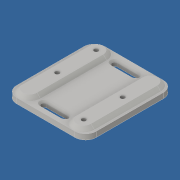
# Autodesk Inventor part: wandler
Saved by Autodesk Inventor 2016 (Build 200138000, 138)
## iProperties
Created: 2015-10-23
Part Number: wandler
Material: Generisch
Document SubType Name: Modeling
Designer: 4ndreas
Density: 1 g/cm^3
Appearance: Vorgabe
Author: 4ndreas
Autodesk Inventor part; units mm, degrees
ref_plane "YZ Plane" through (0, 0, 0) normal (1, 0, 0) x (0, 1, 0)
ref_plane "XZ Plane" through (0, 0, 0) normal (0, 1, 0) x (-1, 0, 0)
ref_plane "XY Plane" through (0, 0, 0) normal (0, 0, 1) x (1, 0, 0)
sketch "Skizze1" plane through (0, 0, 0) normal (0, 0, 1) x (1, 0, 0)
  line L0 (-22.5, -25) -> (22.5, -25)
  line L1 (22.5, -25) -> (22.5, 25)
  line L2 (22.5, 25) -> (-22.5, 25)
  line L3 (-22.5, 25) -> (-22.5, -25)
  line L4 (-22.5, -25) -> (22.5, 25) construction
  line L5 (22.5, -25) -> (-22.5, 25) construction
  line L6 (0, 11) -> (0, -11) construction
  line L7 (-15.25, 18.75) -> (15.25, 18.75) construction
  line L8 (15.25, 18.75) -> (15.25, 3.25) construction
  line L9 (15.25, 3.25) -> (-15.25, 3.25) construction
  line L10 (-15.25, 3.25) -> (-15.25, 18.75) construction
  line L11 (-15.25, 18.75) -> (15.25, 3.25) construction
  line L12 (15.25, 18.75) -> (-15.25, 3.25) construction
  line L13 (-17.7097, 20) -> (17.7097, 20) construction
  line L14 (17.7097, 20) -> (17.7097, 2) construction
  line L15 (17.7097, 2) -> (-17.7097, 2) construction
  line L16 (-17.7097, 2) -> (-17.7097, 20) construction
  line L17 (-17.7097, 20) -> (17.7097, 2) construction
  line L18 (17.7097, 20) -> (-17.7097, 2) construction
  line L19 (-15.25, -18.75) -> (15.25, -18.75) construction
  line L20 (15.25, -18.75) -> (15.25, -3.25) construction
  line L21 (15.25, -3.25) -> (-15.25, -3.25) construction
  line L22 (-15.25, -3.25) -> (-15.25, -18.75) construction
  line L23 (-15.25, -18.75) -> (15.25, -3.25) construction
  line L24 (15.25, -18.75) -> (-15.25, -3.25) construction
  circle A0 centre (-15.25, 18.75) radius 1.25
  circle A1 centre (15.25, 3.25) radius 1.25
  circle A2 centre (15.25, -18.75) radius 1.25
  circle A3 centre (-15.25, -3.25) radius 1.25
  point P0 (0, 0)
  point P1 (0, 0)
  dimension "d0" = 45
  dimension "d1" = 15.5
  dimension "d2" = 30.5
  dimension "d3" = 2
  dimension "d4" = 18
  dimension "d5" = 25
  dimension "d6" = 2.5
  constraints: 50 end point, 10 midpoint, 9 parallel, 7 coincident, 4 centre point, 4 horizontal, 4 perpendicular, 3 equal radius, 3 point on line, 2 equal length
  measures "d0" distance between parallel lines of L3 L1
  measures "d1" distance between parallel lines of L9 L7
  measures "d2" distance between parallel lines of L8 L10
  measures "d3" distance from line of point (0, 0) L15
  measures "d4" distance between parallel lines of L15 L13
  measures "d5" distance from line of point (0, 0) L2
  measures "d6" diameter of A0
extrude "Extrusion1" add sketch "Skizze1" along normal blind 3
fillet "Rundung1" radius 6 4 edges at (-22.5, 25, 1.5) (-22.5, -25, 1.5) (22.5, -25, 1.5) (22.5, 25, 1.5)
chamfer "Fase1" distance 2 angle 45 4 edges at (-16.5, -3.25, 0) (14, -18.75, 0) (14, 3.25, 0) (-16.5, 18.75, 0)
sketch "Skizze2" plane through (0, 0, 3) normal (0, 0, 1) x (1, 0, 0)
  arc A0 (22.5, 19) -> (16.5, 25) centre (16.5, 19) ccw projected
  line L0 (16.5, 25) -> (-16.5, 25) projected
  arc A1 (-16.5, 25) -> (-22.5, 19) centre (-16.5, 19) ccw projected
  line L1 (-22.5, 19) -> (-22.5, -19) projected
  arc A2 (-22.5, -19) -> (-16.5, -25) centre (-16.5, -19) ccw projected
  line L2 (-16.5, -25) -> (16.5, -25) projected
  arc A3 (16.5, -25) -> (22.5, -19) centre (16.5, -19) ccw projected
  line L3 (22.5, -19) -> (22.5, 19) projected
  circle A4 centre (-15.25, -3.25) radius 1.25 projected
  circle A5 centre (15.25, -18.75) radius 1.25 projected
  circle A6 centre (15.25, 3.25) radius 1.25 projected
  circle A7 centre (-15.25, 18.75) radius 1.25 projected
  circle A8 centre (15.25, 3.25) radius 4
  circle A9 centre (15.25, -18.75) radius 4
  circle A10 centre (-15.25, -3.25) radius 4
  circle A11 centre (-15.25, 18.75) radius 4
  line L4 (15.25, -18.75) -> (15.25, 18.75) construction
  line L5 (19.25, -18.75) -> (19.25, 18.75)
  line L6 (11.25, 18.75) -> (11.25, -18.75)
  arc A12 (11.25, -18.75) -> (19.25, -18.75) centre (15.25, -18.75) ccw
  arc A13 (19.25, 18.75) -> (11.25, 18.75) centre (15.25, 18.75) ccw
  line L7 (-15.25, 18.75) -> (-15.25, -18.75) construction
  line L8 (-19.25, 18.75) -> (-19.25, -18.75)
  line L9 (-11.25, -18.75) -> (-11.25, 18.75)
  arc A14 (-11.25, 18.75) -> (-19.25, 18.75) centre (-15.25, 18.75) ccw
  arc A15 (-19.25, -18.75) -> (-11.25, -18.75) centre (-15.25, -18.75) ccw
  line L10 (-15.25, -18.75) -> (15.25, -18.75) construction
  line L11 (15.25, 18.75) -> (-15.25, 18.75) construction
  point P0 (0, 0)
  point P1 (15.25, 0)
  point P2 (-15.25, 0)
  dimension "d13" = 8
  constraints: 21 end point, 9 tangent, 8 centre point, 8 point on circle, 4 coincident, 4 equal radius, 4 parallel, 2 midpoint, 2 perpendicular, 1 vertical
  measures "d13" diameter of A8
extrude "Extrusion2" add sketch "Skizze2" along normal blind 2 contours A8 | L5 A9 L6 A8 | A8 L6 A13 L5 | A9 | A10 | L9 A15 L8 A10 | A10 L8 A11 L9 | A11
chamfer "Fase3" distance 2 angle 45 8 edges at (15.25, 22.75, 3) (19.25, 0, 3) (15.25, -22.75, 3) (11.25, 0, 3) (-15.25, 22.75, 3) (-11.25, 0, 3) (-15.25, -22.75, 3) (-19.25, 0, 3)
sketch "Skizze4" plane through (0, 0, 3) normal (0, 0, 1) x (1, 0, 0)
  line L0 (-6, 20) -> (6, 20) construction
  line L1 (-6, 21.5) -> (6, 21.5)
  line L2 (6, 18.5) -> (-6, 18.5)
  arc A0 (-6, 21.5) -> (-6, 18.5) centre (-6, 20) ccw
  arc A1 (6, 18.5) -> (6, 21.5) centre (6, 20) ccw
  line L3 (-6, -20) -> (6, -20) construction
  line L4 (-6, -18.5) -> (6, -18.5)
  line L5 (6, -21.5) -> (-6, -21.5)
  arc A2 (-6, -18.5) -> (-6, -21.5) centre (-6, -20) ccw
  arc A3 (6, -21.5) -> (6, -18.5) centre (6, -20) ccw
  line L6 (0, -20) -> (0, 20)
  point P0 (0, 0)
  point P1 (0, 0)
  dimension "d22" = 3
  dimension "d23" = 12
  dimension "d24" = 40
  constraints: 18 end point, 8 point on circle, 8 tangent, 4 centre point, 4 parallel, 3 midpoint, 1 coincident, 1 equal radius, 1 horizontal, 1 vertical
  measures "d22" distance between parallel lines of L1 L2
  measures "d23" distance of L0.start L0.end
  measures "d24" distance between parallel lines of L3 L0
extrude "Extrusion3" cut sketch "Skizze4" against normal through all
chamfer "Fase4" distance 1 angle 45 8 edges at (7.5, 20, 3) (0, 18.5, 3) (-7.5, 20, 3) (0, 21.5, 3) (7.5, -20, 3) (0, -21.5, 3) (-7.5, -20, 3) (0, -18.5, 3)
